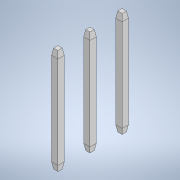
# Autodesk Inventor part: Conector 3 pines
Saved by Autodesk Inventor 2020.3 (Build 243373000, 373)
## iProperties
Created: 2020-06-20
Part Number: Conector 3 pines
Material: Genérico
Document SubType Name: Modeling
Designer: javic
Density: 1 g/cm^3
Appearance: Valor por defecto
Author: javic
Autodesk Inventor part; units mm, degrees
ref_plane "YZ Plane" through (0, 0, 0) normal (1, 0, 0) x (0, 1, 0)
ref_plane "XZ Plane" through (0, 0, 0) normal (0, 1, 0) x (-1, 0, 0)
ref_plane "XY Plane" through (0, 0, 0) normal (0, 0, 1) x (1, 0, 0)
sketch "Boceto1" plane through (0, 0, 0) normal (0, 1, 0) x (-1, 0, 0)
  line L0 (0, 0) -> (0.5, 0)
  line L1 (0.5, 0) -> (0.5, -0.5)
  line L2 (0.5, -0.5) -> (0, -0.5)
  line L3 (0, -0.5) -> (0, 0)
  line L4 (0, -2.54) -> (0.5, -2.54)
  line L5 (0.5, -2.54) -> (0.5, -3.04)
  line L6 (0.5, -3.04) -> (0, -3.04)
  line L7 (0, -3.04) -> (0, -2.54)
  line L8 (0, -5.08) -> (0.5, -5.08)
  line L9 (0.5, -5.08) -> (0.5, -5.58)
  line L10 (0.5, -5.58) -> (0, -5.58)
  line L11 (0, -5.58) -> (0, -5.08)
  dimension "d0" = 0.5
  dimension "d1" = 0.5
  dimension "d2" = 0.5
  dimension "d3" = 0.5
  dimension "d7" = 2.04
  dimension "d8" = 0.5
  dimension "d9" = 0.5
  dimension "d10" = 2.04
  constraints: 24 end point, 6 parallel, 3 horizontal, 3 perpendicular, 1 point on line
  measures "d0" distance of L1.end L2.end
  measures "d1" distance of L0.end L1.end
  measures "d2" distance of L5.end L6.end
  measures "d3" distance of L4.end L5.end
  measures "d7" distance between parallel lines of L2 L4
  measures "d8" distance of L9.end L10.end
  measures "d9" distance of L8.end L9.end
  measures "d10" distance between parallel lines of L6 L8
extrude "Extrusión1" add sketch "Boceto1" along normal blind 8.3
chamfer "Chaflán1" distance 0.08 distance2 0.5 1 edges at (-0.25, 8.3, 0) measured on face at (-0.1667, 8.3, -0.1667)
chamfer "Chaflán2" distance 0.08 distance2 0.5 1 edges at (0, 8.3, -0.29) measured on face at (-0.1667, 8.3, -0.22)
chamfer "Chaflán3" distance 0.08 distance2 0.5 1 edges at (-0.29, 8.3, -0.5) measured on face at (-0.22, 8.3, -0.22)
chamfer "Chaflán4" distance 0.08 distance2 0.5 1 edges at (-0.5, 8.3, -0.25) measured on face at (-0.22, 8.3, -0.1933)
chamfer "Chaflán5" distance 0.08 distance2 0.5 1 edges at (-0.5, 8.3, -2.79) measured on face at (-0.1667, 8.3, -2.7067)
chamfer "Chaflán6" distance 0.08 distance2 0.5 1 edges at (-0.21, 8.3, -2.54) measured on face at (-0.14, 8.3, -2.7067)
chamfer "Chaflán7" distance 0.08 distance2 0.5 1 edges at (-0.21, 8.3, -3.04) measured on face at (-0.14, 8.3, -2.76)
chamfer "Chaflán8" distance 0.08 distance2 0.5 1 edges at (0, 8.3, -2.79) measured on face at (-0.14, 8.3, -2.7333)
chamfer "Chaflán9" distance 0.08 distance2 0.5 1 edges at (-0.5, 8.3, -5.33) measured on face at (-0.1667, 8.3, -5.2467)
chamfer "Chaflán10" distance 0.08 distance2 0.5 1 edges at (-0.21, 8.3, -5.08) measured on face at (-0.14, 8.3, -5.2467)
chamfer "Chaflán11" distance 0.08 distance2 0.5 1 edges at (-0.21, 8.3, -5.58) measured on face at (-0.14, 8.3, -5.3)
chamfer "Chaflán12" distance 0.08 distance2 0.5 1 edges at (0, 8.3, -5.33) measured on face at (-0.14, 8.3, -5.2733)
chamfer "Chaflán13" distance 0.5 distance2 0.08 1 edges at (-0.5, 0, -0.25) measured on face at (-0.5, 2.6, -0.3333)
chamfer "Chaflán14" distance 0.5 distance2 0.08 1 edges at (-0.21, 0, -0.5) measured on face at (-0.1667, 2.7667, -0.5)
chamfer "Chaflán15" distance 0.5 distance2 0.08 1 edges at (0, 0, -0.21) measured on face at (0, 2.7667, -0.1667)
chamfer "Chaflán16" distance 0.5 distance2 0.08 1 edges at (-0.25, 0, 0) measured on face at (-0.3333, 2.9333, 0)
chamfer "Chaflán17" distance 0.5 distance2 0.08 1 edges at (-0.5, 0, -2.79) measured on face at (-0.5, 5.2, -2.7067)
chamfer "Chaflán18" distance 0.5 distance2 0.08 1 edges at (-0.21, 0, -2.54) measured on face at (-0.1667, 2.7667, -2.54)
chamfer "Chaflán19" distance 0.5 distance2 0.08 1 edges at (-0.21, 0, -3.04) measured on face at (-0.1667, 2.7667, -3.04)
chamfer "Chaflán20" distance 0.5 distance2 0.08 1 edges at (0, 0, -2.79) measured on face at (0, 2.9333, -2.7067)
chamfer "Chaflán21" distance 0.5 distance2 0.08 1 edges at (-0.5, 0, -5.33) measured on face at (-0.5, 5.2, -5.2467)
chamfer "Chaflán22" distance 0.5 distance2 0.08 1 edges at (-0.21, 0, -5.08) measured on face at (-0.1667, 2.7667, -5.08)
chamfer "Chaflán23" distance 0.5 distance2 0.08 1 edges at (0, 0, -5.37) measured on face at (0, 2.7667, -5.4133)
chamfer "Chaflán24" distance 0.5 distance2 0.08 1 edges at (-0.25, 0, -5.58) measured on face at (-0.1667, 2.9333, -5.58)
